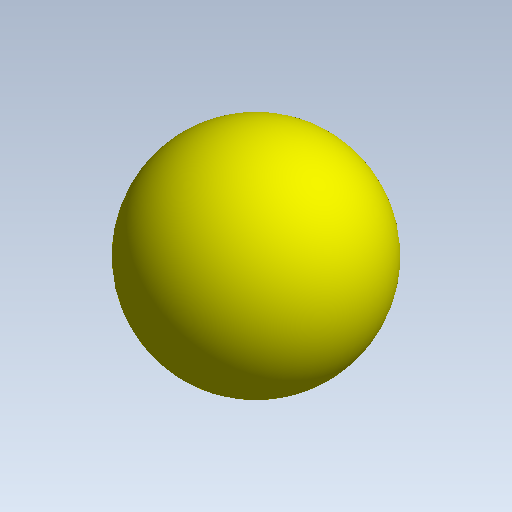
# Autodesk Inventor part: W 61700 X-2RS1_PART3
Saved by Autodesk Inventor 2021 (Build 250183000, 183)
## iProperties
Part Number: W 61700 X-2RS1_PART3
Material: Allgemein
Catalog Web Link: www.cadenas.de
Description: -Deep groove ball bearings
Vendor: SKF
Document SubType Name: Modeling
Designer: partserver
Manufacturer: SKF
Mass: 0.00209677 g
Surface Area: 0.0792229 cm^2
Volume: 0.00209677 cm^3
Density: 1 g/cm^3
Appearance: PSOLRGB-192-192-192
Category: PARTsolutions
Company: SKF
PSOL_IDENT_0: {$CADENAS_DATA\23d-libs\skf_r32\bearings_units_and_housings\ball_bearings\deep_groove_ball_bearings\
PSOL_IDENT_1: bb1_001_101.prj},207 {VTYP=3D},{NB=W 61700 X-2RS1_PART3},{LINA=W 61700 X-2RS1_PART3},{NN=BB1_001_101
PSOL_IDENT_2: _PART3},{NOPRJ=TRUE},{DATE=12.05.2020 07:47:22},{GEOMDATE=07.04.2020 07:08:50},{VERSION=},{LINEID=18
PSOL_IDENT_3: 530},{WBVAR=},{WBNUMERIC=}  {NB=W 61700 X-2RS1_PART3},{LINA=W 61700 X-2RS1_PART3},{KT=DUMMY},{DESIGN
PSOL_IDENT_4: ATION=W 61700 X-2RS1},{DD=10.000},{D=15.000},{B=4.000},{C=0.000},{DD1=11.21},{DD2=0.00},{D1=0.00},{D
PSOL_IDENT_5: 2=14.20},{D3=0.000},{D4=0.000},{HH=MIN},{BB=0.000},{FF=0.00},{R0MAX=MIN},{R0=MIN},{R12=0.15},{PITCH=
PSOL_IDENT_6: 12.49},{DW=1.588},{DDAMIN=11.000},{DDAMAX=11.000},{DDBMIN=MIN},{DDBMAX=MIN},{DBMIN=MIN},{DAMAX=14.50
PSOL_IDENT_7: 0},{BBAMIN=MIN},{CAMAX=MIN},{RAMAX=0.150},{LOAD1=0.488},{LOAD2=0.220},{LOAD3=0.009},{SPEED1=MIN},{SP
PSOL_IDENT_8: EED2=24000},{KR=0.015},{F0=8.000},{Z=11},{II=1},{MASS=0.002},{BEARING=W 61700 X-2RS1},{RING=},{HELP=
PSOL_IDENT_9: 0.723},{HELP2=0.400},{DD1ALG=5.605},{YALG=5.605},{PITCH1=12.490},{DW1=1.588},{YALG1=6.777},{HALG1=0.
PSOL_IDENT_10: 723},{SH=5.605},{CU=0.482},{DESIGN=dgbbw2rs},{HALG=0.605},{B1=0},{SHIELDHELP=2}
NB: W 61700 X-2RS1_PART3
NT: Deep groove ball bearings
NBSYN: $DESIGNATION._PART3
LINA: W 61700 X-2RS1_PART3
CATALOG: SKF
SUPPLIER: SKF
ARTICLENO: W 61700 X-2RS1_PART3
BOMINFO: W 61700 X-2RS1_PART3
CREATOR: CADENAS GmbH
Title: W 61700 X-2RS1_PART3
Author: Cadenas PARTsolutions
Comments: Deep groove ball bearings
Autodesk Inventor part; units mm, degrees
ref_plane "YZ Plane" through (0, 0, 0) normal (1, 0, 0) x (0, 1, 0)
ref_plane "XZ Plane" through (0, 0, 0) normal (0, 1, 0) x (-1, 0, 0)
ref_plane "XY Plane" through (0, 0, 0) normal (0, 0, 1) x (1, 0, 0)
sketch "Sketch_6" plane through (0, 0, 0) normal (0, 0, 1) x (1, 0, 0)
  line L0 (2.794, 6.245) -> (1.206, 6.245)
  arc A0 (2.794, 6.245) -> (1.206, 6.245) centre (2, 6.245) ccw
  line L1 (2.794, 6.245) -> (1.206, 6.245)
  dimension "d0" = 360
  constraints: 4 end point, 2 point on circle, 1 centre point
revolve "Revolution1" add sketch "Sketch_6" angle 360 about axis through (2.794, 6.245, 0) along (1, 0, 0)
body "Solid1"
